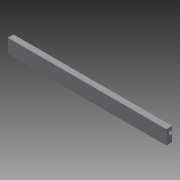
# Autodesk Inventor part: bottom_board_side_slat
Saved by Autodesk Inventor 2014 SP1 (Build 180222100, 222)
## iProperties
Created: 2014-02-20
Part Number: bottom_board_side_slat
Material: Wood (Birch)
Document SubType Name: Modeling
Designer: Chris
Density: 0.55 g/cm^3
Appearance: Birch - Natural Polished
Mass: 239.546 g
Surface Area: 829.232 cm^2
Volume: 435.537 cm^3
Author: Chris
Autodesk Inventor part; units mm, degrees
ref_plane "YZ Plane" through (0, 0, 0) normal (1, 0, 0) x (0, 1, 0)
ref_plane "XZ Plane" through (0, 0, 0) normal (0, 1, 0) x (-1, 0, 0)
ref_plane "XY Plane" through (0, 0, 0) normal (0, 0, 1) x (1, 0, 0)
sketch "Sketch1" plane through (0, 0, 0) normal (0, 0, 1) x (1, 0, 0)
  line L0 (0, 0) -> (-533.4, 0)
  line L1 (-533.4, 0) -> (-533.4, 47.625)
  line L2 (-533.4, 47.625) -> (0, 47.625)
  line L3 (0, 47.625) -> (0, 0)
  dimension "d0" = 533.4
  dimension "d1" = 47.625
  dimension "d2" = 0
  dimension "d3" = 0
  constraints: 8 end point, 2 parallel, 1 horizontal, 1 perpendicular
  measures "d0" distance of L1.end L2.end
  measures "d1" distance of L0.end L1.end
  measures "d2" distance from line of point (0, 0) L0
  measures "d3" distance from line of L3 point (0, 0)
extrude "Extrusion1" add sketch "Sketch1" against normal blind 19.05
sketch "Sketch2" plane through (0, 0, 0) normal (1, 0, 0) x (0, 0, -1)
  line L0 (0, 0) -> (19.05, 0) projected
  line L1 (0, 47.625) -> (19.05, 47.625)
  line L2 (19.05, 47.625) -> (19.05, 0)
  line L3 (19.05, 0) -> (0, 0)
  line L4 (0, 0) -> (0, 47.625)
  line L5 (19.05, 34.925) -> (9.525, 34.925)
  line L6 (9.525, 34.925) -> (9.525, 25.4)
  line L7 (9.525, 25.4) -> (19.05, 25.4)
  line L8 (19.05, 25.4) -> (19.05, 34.925)
  dimension "d6" = 12.7
  dimension "d7" = 9.525
  dimension "d8" = 25.4
  dimension "d11" = 9.525
  constraints: 16 end point, 4 parallel, 2 horizontal, 2 perpendicular, 1 point on line
  measures "d6" distance between parallel lines of L1 L5
  measures "d7" distance of L5.end L6.end
  measures "d8" distance between parallel lines of L0 L7
  measures "d11" distance of L5.start L5.end
extrude "Extrusion2" cut sketch "Sketch2" against normal through all contours L7 L6 L5 L2
body "Solid1"
